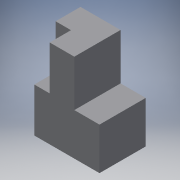
# Autodesk Inventor part: part_b
Saved by Autodesk Inventor 2019 (Build 230136000, 136)
## iProperties
Created: 2019-01-14
Part Number: part_b
Material: Generic
Document SubType Name: Modeling
Designer: jmc
Density: 1 g/cm^3
Appearance: Default
Author: jmc
Autodesk Inventor part; units mm, degrees
ref_plane "YZ Plane" through (0, 0, 0) normal (1, 0, 0) x (0, 1, 0)
ref_plane "XZ Plane" through (0, 0, 0) normal (0, 1, 0) x (-1, 0, 0)
ref_plane "XY Plane" through (0, 0, 0) normal (0, 0, 1) x (1, 0, 0)
sketch "Sketch1" plane through (0, 0, 0) normal (0, 0, 1) x (1, 0, 0)
  line L0 (-13.4791, 11.2201) -> (28.8409, 11.2201)
  line L1 (28.8409, 11.2201) -> (28.8409, -16.0394)
  line L2 (28.8409, -16.0394) -> (-13.4791, -16.0394)
  line L3 (-13.4791, -16.0394) -> (-13.4791, 11.2201)
  point P0 (0, 0)
  constraints: 8 end point, 2 parallel, 1 horizontal, 1 perpendicular
extrude "Extrusion1" add sketch "Sketch1" against normal blind 30
sketch "Sketch2" plane through (-13.4791, 11.2201, 0) normal (0, 1, 0) x (1, 0, 0)
  line L0 (0, 30) -> (42.32, 30) projected
  line L1 (0, 0) -> (42.32, 0) projected
  line L2 (0, 30) -> (25.9794, 30)
  line L3 (25.9794, 30) -> (25.9794, 0)
  line L4 (25.9794, 0) -> (0, 0)
  line L5 (0, 0) -> (0, 30)
  point P0 (13.4791, 0)
  constraints: 8 end point, 2 parallel, 1 horizontal, 1 perpendicular, 1 point on line
extrude "Extrusion2" add sketch "Sketch2" along normal blind 30
sketch "Sketch3" plane through (-13.4791, -16.0394, -30) normal (-1, 0, 0) x (0, 0, 1)
  line L0 (0, 57.2595) -> (30, 57.2595) projected
  line L1 (30, 0) -> (30, 57.2595) projected
  line L2 (16.1769, 57.2595) -> (30, 57.2595)
  line L3 (30, 57.2595) -> (30, 28.6298)
  line L4 (30, 28.6298) -> (16.1769, 28.6298)
  line L5 (16.1769, 28.6298) -> (16.1769, 57.2595)
  point P0 (30, 16.0394)
  constraints: 8 end point, 2 parallel, 1 horizontal, 1 midpoint, 1 perpendicular, 1 point on line
extrude "Extrusion3" cut sketch "Sketch3" against normal blind 10
body "Solid1"
